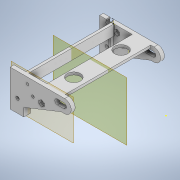
# Autodesk Inventor part: Capping_RotatingArm
Saved by Autodesk Inventor 2022 (Build 260153000, 153)
## iProperties
Created: 2024-05-06
Part Number: Capping_RotatingArm
Material: Generic
Document SubType Name: Modeling
Designer: Gotham City
Density: 1 g/cm^3
Appearance: Default
Author: Gotham City
Autodesk Inventor part; units mm, degrees
ref_plane "YZ Plane" through (0, 0, 0) normal (1, 0, 0) x (0, 1, 0)
ref_plane "XZ Plane" through (0, 0, 0) normal (0, 1, 0) x (-1, 0, 0)
ref_plane "XY Plane" through (0, 0, 0) normal (0, 0, 1) x (1, 0, 0)
sketch "Sketch1" plane through (0, 0, 0) normal (0, 0, 1) x (1, 0, 0)
  line L0 (-11.7769, 40.6389) -> (-42.4029, 40.6389) construction
  line L1 (-41.8029, 32.9379) -> (-41.8029, 12.9379) projected
  line L2 (-11.7769, 35.6389) -> (-42.4029, 35.6389) construction
  circle A0 centre (-45.1029, 22.9379) radius 1.3 projected
  point P0 (0, 0)
sketch "Sketch3" plane through (0, 0, 0) normal (0, 0, 1) x (1, 0, 0)
  line L0 (-41.8029, 32.9379) -> (-41.8029, 12.9379) construction
  line L1 (-41.8029, 12.9379) -> (-50.8029, 12.9379)
  line L2 (-50.8029, 12.9379) -> (-50.8029, 32.9379)
  line L3 (-50.8029, 32.9379) -> (-41.8029, 32.9379)
  line L4 (-41.8029, 32.9379) -> (-41.8029, 12.9379)
  line L5 (-50.8029, 22.9379) -> (-41.8029, 22.9379) construction
  circle A0 centre (-45.1029, 22.9379) radius 1.3
  line L6 (-11.7769, 40.6389) -> (-41.8029, 40.6389)
  line L7 (-41.8029, 40.6389) -> (-41.8029, 30.6389)
  line L8 (-41.8029, 30.6389) -> (-11.7769, 30.6389)
  line L9 (-11.7769, 30.6389) -> (-11.7769, 40.6389)
  line L10 (-11.7769, 40.6389) -> (-41.8029, 30.6389) construction
  line L11 (-41.8029, 40.6389) -> (-11.7769, 30.6389) construction
  line L12 (-42.4029, 35.6389) -> (-11.7769, 35.6389) construction
  line L13 (-11.7769, 40.6389) -> (-42.4029, 40.6389) construction
  circle A1 centre (-11.7769, 35.6389) radius 1.5 construction
  line L14 (-50.8029, 40.6389) -> (-11.7769, 40.6389)
  line L15 (-11.7769, 40.6389) -> (-9.2769, 40.6389)
  line L16 (-11.7769, 35.6389) -> (-9.7769, 35.6389) construction
  line L17 (-14.7769, 33.6889) -> (-9.7769, 33.6889)
  line L18 (-9.7769, 37.5889) -> (-14.7769, 37.5889)
  arc A2 (-9.7769, 33.6889) -> (-9.7769, 37.5889) centre (-9.7769, 35.6389) ccw
  line L19 (-11.7769, 30.6389) -> (-9.2769, 30.6389)
  arc A3 (-9.2769, 30.6389) -> (-9.2769, 40.6389) centre (-9.2769, 35.6389) ccw
  arc A4 (-14.7769, 37.5889) -> (-14.7769, 33.6889) centre (-14.7769, 35.6389) ccw
  circle A5 centre (-45.1029, 22.9379) radius 1.3 construction
  line L20 (-14.7769, 35.6389) -> (-11.7769, 35.6389) construction
  line L21 (-50.8029, 40.6389) -> (-50.8029, 32.9379)
  line L22 (-11.7769, 30.6389) -> (-41.8029, 18.7521)
  point P0 (0, 0)
  point P1 (-26.7899, 35.6389)
  point P2 (-41.8029, 30.5135)
  point P3 (-11.7769, 34.1389)
  point P4 (-11.7769, 37.1389)
  point P5 (-10.7769, 35.6389)
  dimension "d0" = 9
  dimension "d1" = 5
  dimension "d2" = 0
  dimension "d3" = 3
  dimension "d45" = 3.9
  dimension "d46" = 2
  dimension "d48" = 7.5
  dimension "d65" = 3
  dimension "d91" = 2.6
  dimension "d112" = 11.8868
  constraints: 45 end point, 6 midpoint, 6 parallel, 6 point on circle, 6 tangent, 5 centre point, 4 coincident, 4 point on line, 3 collinear, 3 horizontal, 3 perpendicular
  measures "d0" distance of L2.end L3.end
  measures "d1" distance between parallel lines of L8 L12
  measures "d2" distance between parallel lines of L6 L13
  measures "d3" diameter of A1
  measures "d45" distance between parallel lines of L17 L18
  measures "d46" distance of L16.start L16.end
  measures "d65" distance of L20.start L12.end
  measures "d91" diameter of A0
  measures "d112" distance from line of L8 L22.end
extrude "Extrusion1" add sketch "Sketch3" against normal blind 3 contours L1 L2 L3 L4 | L4 L8 L22 | L21 L14 L7 L3 | L4 L7 L6 L9 L18 A4 L17 L8 | L9 L17 A2 L18 L15 A3 L19
ref_plane "Work Plane2" through (0, 0, 32.5) normal (0, 0, 1) x (1, 0, 0)
ref_plane "Work Plane1" through (0, 0, 65) normal (0, 0, 1) x (1, 0, 0)
sketch "Sketch12" plane through (0, 0, -3) normal (0, 0, 1) x (1, 0, 0)
  line L0 (-41.8029, 18.7521) -> (-41.8029, 12.9379) projected
  line L1 (-41.8029, 12.9379) -> (-41.8029, 40.6389)
  line L2 (-41.8029, 40.6389) -> (-40.3029, 40.6389)
  line L3 (-40.3029, 40.6389) -> (-40.3029, 12.9379)
  line L4 (-40.3029, 12.9379) -> (-41.8029, 12.9379)
  line L5 (-9.2769, 40.6389) -> (-50.8029, 40.6389) projected
  point P0 (0, 0)
  point P1 (-41.8029, 22.9379)
  point P2 (-41.8029, 22.9379)
  point P3 (-41.8029, 30.6389)
  dimension "d50" = 1.5
  constraints: 8 end point, 2 point on line, 1 collinear, 1 parallel, 1 perpendicular
  measures "d50" distance between parallel lines of L3 L0
extrude "Extrusion9" add sketch "Sketch12" along normal blind 5
thicken "Thicken3" operation add thickness 0.1 both sides no extend neighbours yes toward (1, 0, 0) faces at (-41.8029, 31.4052, 0.6667)
mirror "Mirror1" about plane through (0, 0, 32.5) normal (0, 0, 1) of "Extrusion1", "Extrusion9", "Thicken3"
sketch "Sketch4" plane through (0, 0, 0) normal (0, 0, 1) x (1, 0, 0)
  line L0 (-11.7769, 40.6389) -> (-11.7769, 38.6389)
  line L1 (-11.7769, 40.6389) -> (-42.4029, 40.6389) construction
  line L2 (-11.7769, 38.6389) -> (-25.7769, 38.6389)
  line L3 (-25.7769, 38.6389) -> (-25.7769, 40.6389)
  line L4 (-11.7769, 40.6389) -> (-25.7769, 40.6389)
  point P0 (0, 0)
  point P1 (-14.4207, 40.1217)
  dimension "d8" = 2
  dimension "d9" = 14
  constraints: 8 end point, 2 perpendicular, 1 parallel, 1 point on line
  measures "d8" distance of L0.start L0.end
  measures "d9" distance of L0.end L2.end
extrude "Extrusion2" add sketch "Sketch4" along normal up to surface (65 mm away)
sketch "Sketch10" plane through (-25.7769, 38.6389, 0) normal (0, -1, 0) x (1, 0, 0)
  line L0 (14, 0) -> (14, 65) construction
  line L1 (0, 0) -> (0, 65) construction
  circle A0 centre (6, 14.5) radius 5.025
  line L2 (-39.1518, 32.5) -> (36.5984, 32.5) projected
  point P0 (25.7769, 0)
  point P1 (5.5291, 32.5)
  dimension "d25" = 10.05
  dimension "d28" = 8
  dimension "d68" = 18
  constraints: 1 centre point, 1 point on line
  measures "d25" diameter of A0
  measures "d28" distance from line of A0.centre L0
  measures "d68" vertical distance of A0.centre point (5.529, 32.5)
extrude "Extrusion8" cut sketch "Sketch10" against normal blind 2.55
sketch "Sketch16" plane through (0, 0, 0) normal (0, 0, 1) x (1, 0, 0)
  line L0 (-39.7029, 40.6389) -> (-39.7029, 32.6534)
  line L1 (-39.7029, 32.6534) -> (-41.7029, 32.6534)
  line L2 (-41.7029, 40.6389) -> (-41.7029, 12.9379) projected
  line L3 (-41.7029, 40.6389) -> (-39.7029, 40.6389)
  line L4 (-41.7029, 32.6534) -> (-41.7029, 40.6389)
  point P0 (0, 0)
  point P1 (-40.3029, 40.6389)
  dimension "d62" = 2
  constraints: 8 end point, 2 point on line, 1 collinear, 1 parallel, 1 vertical
  measures "d62" distance between parallel lines of L2 L0
extrude "Extrusion12" add sketch "Sketch16" along normal up to surface (65 mm away)
mirror "Mirror2" about plane through (0, 0, 32.5) normal (0, 0, 1) of "Extrusion8"
sketch "Sketch18" plane through (0, 0, -3) normal (0, 0, -1) x (-1, 0, 0)
  circle A0 centre (32.8063, 30.0277) radius 1 construction
  line L0 (50.8029, 12.9379) -> (50.8029, 40.6389) construction
  circle A1 centre (34.5371, 36.8103) radius 1 construction
  circle A2 centre (45.1029, 22.9379) radius 1.3 construction
  circle A3 centre (45.1029, 22.9379) radius 2.25 construction
  line L1 (28.5428, 23.6333) -> (33.859, 44.4657) construction
  line L2 (33.859, 44.4657) -> (44.2267, 41.82) construction
  line L3 (44.2267, 41.82) -> (38.9105, 20.9876) construction
  line L4 (38.9105, 20.9876) -> (28.5428, 23.6333) construction
  line L5 (54.1073, 49.8023) -> (45.3305, 15.409) construction
  line L6 (34.5371, 36.8103) -> (32.8063, 30.0277) construction
  line L7 (31.2009, 34.0495) -> (41.5686, 31.4038) construction
  circle A4 centre (48.3029, 37.1676) radius 2.5 construction
  line L8 (32.8063, 30.0277) -> (32.9623, 30.6389) construction
  line L9 (11.7769, 30.6389) -> (9.2769, 30.6389) construction
  line L10 (34.5371, 36.8103) -> (34.3812, 36.1991) construction
  line L11 (50.8029, 40.6389) -> (9.2769, 40.6389) projected
  point P0 (0, 0)
  point P1 (33.6717, 33.419)
  dimension "d69" = 2
  dimension "d71" = 7
  dimension "d78" = 4.5
  dimension "d79" = 14.316
  dimension "d80" = 21.5
  dimension "d82" = 10.7
  dimension "d83" = 18.3
  dimension "d84" = 2.55
  dimension "d85" = 5
  dimension "d86" = 3.5
  dimension "d124" = 3.8286
  constraints: 20 end point, 4 centre point, 4 coincident, 4 parallel, 3 midpoint, 3 point on line, 2 collinear, 2 tangent, 1 equal radius, 1 perpendicular
  measures "d69" diameter of A0
  measures "d71" distance of L6.start L6.end
  measures "d78" diameter of A3
  measures "d79" angle of L0 L5
  measures "d80" distance of L1.start L1.end
  measures "d82" distance of L1.end L2.end
  measures "d83" distance between parallel lines of L1 L5
  measures "d84" distance from line of L1 L6.end
  measures "d85" diameter of A4
  measures "d86" distance from line of L2 A4.centre
  measures "d124" distance from line of L11 L6.start
sketch "Sketch19" plane through (0, 0, -3) normal (0, 0, -1) x (-1, 0, 0)
  line L0 (35.7131, 29.2859) -> (29.8994, 30.7695) construction
  line L1 (35.4659, 28.3169) -> (29.6522, 29.8005) construction
  line L2 (30.1467, 31.7384) -> (35.9604, 30.2548) construction
  arc A0 (35.4659, 28.3169) -> (35.9604, 30.2548) centre (35.7131, 29.2859) ccw construction
  arc A1 (30.1467, 31.7384) -> (29.6522, 29.8005) centre (29.8994, 30.7695) ccw construction
  line L3 (34.5371, 36.8103) -> (32.8063, 30.0277) construction
  line L4 (31.2009, 34.0495) -> (41.5686, 31.4038) construction
  line L5 (37.444, 36.0685) -> (31.6303, 37.5521) construction
  line L6 (37.6912, 37.0375) -> (31.8776, 38.5211) construction
  line L7 (31.383, 36.5832) -> (37.1967, 35.0996) construction
  arc A2 (37.1967, 35.0996) -> (37.6912, 37.0375) centre (37.444, 36.0685) ccw construction
  arc A3 (31.8776, 38.5211) -> (31.383, 36.5832) centre (31.6303, 37.5521) ccw construction
  circle A4 centre (32.8063, 30.0277) radius 1 construction
  circle A5 centre (37.444, 36.0685) radius 1
  circle A6 centre (33.3877, 29.8793) radius 1
  point P0 (0, 0)
  dimension "d87" = 2
  dimension "d88" = 6
  dimension "d100" = 0.6
  constraints: 16 end point, 8 point on circle, 6 centre point, 6 symmetric about line, 5 tangent, 1 coincident, 1 concentric, 1 midpoint, 1 parallel, 1 perpendicular, 1 point on line, 2 other
  measures "d87" distance between parallel lines of L2 L1
  measures "d88" distance of L0.start L0.end
  measures "d100" distance of A4.centre A6.centre
extrude "Extrusion13" cut sketch "Sketch19" against normal up to surface (71 mm away)
thicken "Thicken4" operation add thickness 0.1 both sides no extend neighbours yes toward (0, 0, 1) faces at (-45.9218, 35.1687, 65)
thicken "Thicken5" operation add thickness 0.1 both sides no extend neighbours yes toward (0, 0, -1) faces at (-45.9218, 35.1687, 0)
sketch "Sketch20" plane through (0, 0, 0) normal (0, 0, 1) x (1, 0, 0)
  line L0 (-33.3877, 32.2176) -> (-31.3627, 31.0485)
  line L1 (-31.3627, 31.0485) -> (-31.3627, 28.7102)
  line L2 (-31.3627, 28.7102) -> (-33.3877, 27.5411)
  line L3 (-33.3877, 27.5411) -> (-35.4127, 28.7102)
  line L4 (-35.4127, 28.7102) -> (-35.4127, 31.0485)
  line L5 (-35.4127, 31.0485) -> (-33.3877, 32.2176)
  line L6 (-39.469, 34.8994) -> (-39.469, 37.2377)
  line L7 (-39.469, 37.2377) -> (-37.444, 38.4068)
  line L8 (-37.444, 38.4068) -> (-35.419, 37.2377)
  line L9 (-35.419, 37.2377) -> (-35.419, 34.8994)
  line L10 (-35.419, 34.8994) -> (-37.444, 33.7303)
  line L11 (-37.444, 33.7303) -> (-39.469, 34.8994)
  circle A0 centre (-37.444, 36.0685) radius 1 construction
  circle A1 centre (-33.3877, 29.8793) radius 1 construction
  point P0 (0, 0)
  point P1 (-32.7372, 30.6389)
  point P2 (-34.0381, 30.6389)
  dimension "d96" = 4.05
  dimension "d97" = 4.05
  constraints: 24 end point, 2 coincident, 1 parallel, 1 vertical, 26 other
  measures "d96" distance between parallel lines of L5 L2
  measures "d97" distance between parallel lines of L11 L8
extrude "Extrusion14" cut sketch "Sketch20" against normal blind 1.6
mirror "Mirror3" about plane through (0, 0, 32.5) normal (0, 0, 1) of "Extrusion14"
sketch "Sketch21" plane through (0, 0, -3) normal (0, 0, -1) x (-1, 0, 0)
  line L0 (42.2029, 40.6389) -> (45.7029, 40.6389)
  line L1 (42.2029, 40.6389) -> (42.2029, 39.6217)
  arc A0 (42.2029, 39.6217) -> (45.7029, 39.6217) centre (43.9529, 38.6534) ccw
  line L2 (45.7029, 39.6217) -> (45.7029, 40.6389)
  line L3 (40.3029, 12.9379) -> (40.3029, 19.3459) projected
  line L4 (41.7029, 32.6534) -> (41.7029, 12.9379) projected
  line L5 (41.7029, 12.9379) -> (41.7029, 40.6389) projected
  line L6 (41.7029, 12.9379) -> (41.7029, 40.6389) projected
  line L7 (41.7029, 32.6534) -> (41.7029, 12.9379) projected
  line L8 (41.7029, 32.6534) -> (40.3029, 32.6534) projected
  line L9 (40.3029, 32.6534) -> (41.7029, 32.6534) projected
  line L10 (39.7029, 32.6534) -> (40.3029, 32.6534) projected
  line L11 (40.3029, 32.6534) -> (39.7029, 32.6534) projected
  point P0 (0, 0)
  point P1 (40.3029, 23.3226)
  point P2 (40.3029, 30.6389)
  dimension "d105" = 3.5
  dimension "d106" = 2
  dimension "d108" = 0.5
  dimension "d109" = 6
  constraints: 6 end point, 2 point on circle, 2 vertical, 1 centre point, 1 parallel
  measures "d105" distance between parallel lines of L2 L1
  measures "d106" radius of A0
  measures "d108" distance between parallel lines of L5 L1
  measures "d109" distance from line of L8 A0.centre
extrude "Extrusion15" cut sketch "Sketch21" against normal up to surface (2.9 mm away)
sketch "Sketch22" plane through (0, 0, 0) normal (0, 0, 1) x (1, 0, 0)
  circle A0 centre (-26.7769, 28.6389) radius 2 construction
  point P0 (0, 0)
sketch "Sketch23" plane through (0, 0, 0) normal (0, 0, 1) x (1, 0, 0)
  point P0 (0, 0)
  point P1 (-26.7769, 28.6389)
hole "Hole1" at (-26.7769, 28.6389, 0) direction (0, 0, -1) diameter 2.1 depth 12 tip angle 118 clearance for "Socket Head Cap Screw ISO 4762" size "M2" standard "ISO"
sketch "Sketch24" plane through (0, 0, -3) normal (0, 0, -1) x (-1, 0, 0)
  line L0 (28.8269, 29.8225) -> (28.8269, 27.4553)
  line L1 (28.8269, 27.4553) -> (26.7769, 26.2717)
  line L2 (26.7769, 26.2717) -> (24.7269, 27.4553)
  line L3 (24.7269, 27.4553) -> (24.7269, 29.8225)
  line L4 (24.7269, 29.8225) -> (26.7769, 31.006)
  line L5 (26.7769, 31.006) -> (28.8269, 29.8225)
  point P0 (0, 0)
  point P1 (26.7769, 28.6389)
  point P2 (26.7769, 28.6389)
  dimension "d121" = 4.1
  constraints: 12 end point, 1 coincident, 1 vertical, 13 other
  measures "d121" distance between parallel lines of L0 L3
extrude "Extrusion16" cut sketch "Sketch24" against normal blind 1.6
mirror "Mirror4" about plane through (0, 0, 32.5) normal (0, 0, 1) of "Extrusion16", "Hole1"
ref_plane "Work Plane3" through (0, 0, 32.5) normal (0, 0, 1) x (1, 0, 0)
equation "\"d4\" = d3"
equation "\"d10\" = d3"
body "Solid1"
